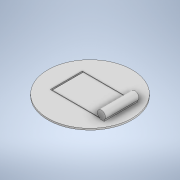
# Autodesk Inventor part: 平板架
Saved by Autodesk Inventor 2021 (Build 250183000, 183)
## iProperties
Created: 2023-03-08
Part Number: 平板架
Material: 一般
Document SubType Name: Modeling
Designer: brian
Density: 1 g/cm^3
Appearance: 預設
Author: brian
Autodesk Inventor part; units mm, degrees
ref_plane "YZ Plane" through (0, 0, 0) normal (1, 0, 0) x (0, 1, 0)
ref_plane "XZ Plane" through (0, 0, 0) normal (0, 1, 0) x (-1, 0, 0)
ref_plane "XY Plane" through (0, 0, 0) normal (0, 0, 1) x (1, 0, 0)
sketch "草圖1" plane through (0, 0, 0) normal (0, 1, 0) x (-1, 0, 0)
  circle A0 centre (0, 0) radius 73
  dimension "d0" = 146
  constraints: 1 centre point, 1 coincident
  measures "d0" diameter of A0
extrude "擠出1" add sketch "草圖1" along normal blind 2.8
sketch "草圖2" plane through (0, 0, 0) normal (0, 0, 1) x (1, 0, 0)
  circle A0 centre (48.9, 10.6) radius 7
  line L0 (73, 0) -> (-73, 0) projected
  line L1 (73, 0) -> (73, 2.8) projected
  line L2 (53.4727, 5.3) -> (53.4727, 2.8)
  line L3 (73, 2.8) -> (-73, 2.8) projected
  line L4 (45.8488, 4.3) -> (45.8488, 2.8)
  point P0 (0, 0)
  point P1 (48.9, 17.6)
  point P2 (41.9, 10.6)
  dimension "d3" = 14
  dimension "d4" = 17.6
  dimension "d5" = 31.1
  dimension "d6" = 1.5
  dimension "d7" = 2.5
  constraints: 4 end point, 4 point on circle, 2 point on line, 1 centre point, 1 horizontal alignment, 1 parallel, 1 vertical, 1 vertical alignment
  measures "d3" diameter of A0
  measures "d4" distance from line of L0 A0.start
  measures "d5" distance from line of L1 A0.end
  measures "d6" distance of L4.start L4.end
  measures "d7" distance of L2.start L2.end
extrude "擠出2" add sketch "草圖2" along normal mid plane 58
sketch "草圖3" plane through (0, 2.8, 0) normal (0, 1, 0) x (1, 0, 0)
  line L0 (-41.1, 27.85) -> (45.8488, 27.85)
  line L1 (45.8488, 27.85) -> (45.8488, -27.85)
  line L2 (45.8488, -27.85) -> (-41.1, -27.85)
  line L3 (-41.1, -27.85) -> (-41.1, 27.85)
  line L4 (-38.6, 26.9) -> (45.8488, 26.9)
  line L5 (45.8488, 26.9) -> (45.8488, -26.9)
  line L6 (45.8488, -26.9) -> (-38.6, -26.9)
  line L7 (-38.6, -26.9) -> (-38.6, 26.9)
  line L8 (45.8488, -29) -> (45.8488, 29) projected
  line L9 (41.9, 29) -> (41.9, -29) projected
  point P0 (0, 0)
  point P1 (-38.6, 0)
  point P2 (-41.1, 0)
  point P3 (41.9, -27.85)
  point P4 (41.9, -26.9)
  point P5 (41.9, 26.9)
  point P6 (41.9, 27.85)
  dimension "d10" = 55.7
  dimension "d11" = 53.8
  dimension "d12" = 80.5
  dimension "d13" = 83
  constraints: 16 end point, 4 parallel, 2 collinear, 2 horizontal, 2 horizontal alignment, 2 midpoint, 2 perpendicular
  measures "d10" distance of L2.end L0.start
  measures "d11" distance of L6.end L4.start
  measures "d12" distance between parallel lines of L9 L7
  measures "d13" distance between parallel lines of L9 L3
extrude "擠出3" cut sketch "草圖3" against normal through all contours L0 L9 L4 L7 L6 L2 L3 | L0 L1 L4 L9 | L9 L6 L1 L2
